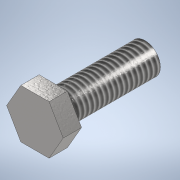
# Autodesk Inventor part: Болт
Saved by Autodesk Inventor 2023 (Build 270158000, 158)
## iProperties
Created: 2022-10-30
Part Number: Болт
Material: Типовые
Document SubType Name: Modeling
Designer: Admin
Density: 1 g/cm^3
Appearance: По умолчанию
Author: Admin
Autodesk Inventor part; units mm, degrees
ref_plane "YZ Plane" through (0, 0, 0) normal (1, 0, 0) x (0, 1, 0)
ref_plane "XZ Plane" through (0, 0, 0) normal (0, 1, 0) x (-1, 0, 0)
ref_plane "XY Plane" through (0, 0, 0) normal (0, 0, 1) x (1, 0, 0)
sketch "Эскиз1" plane through (0, 0, 0) normal (0, 0, 1) x (1, 0, 0)
  line L0 (2.3094, 4) -> (4.6188, 0)
  line L1 (4.6188, 0) -> (2.3094, -4)
  line L2 (2.3094, -4) -> (-2.3094, -4)
  line L3 (-2.3094, -4) -> (-4.6188, 0)
  line L4 (-4.6188, 0) -> (-2.3094, 4)
  line L5 (-2.3094, 4) -> (2.3094, 4)
  circle A0 centre (0, 0) radius 2.5
  dimension "d0" = 8
  dimension "d3" = 5
  constraints: 12 end point, 2 coincident, 1 centre point, 1 horizontal, 13 other
  measures "d0" distance between parallel lines of L2 L5
  measures "d3" diameter of A0
extrude "Выдавливание1" add sketch "Эскиз1" along normal blind 3 contours L0 L1 L2 L3 L4 L5 | A0
extrude "Выдавливание2" add sketch "Эскиз1" against normal blind 15 contours A0
thread "Резьба1" size "M5x0.8" class "6g" standard "ISO Metric profile" length 150
